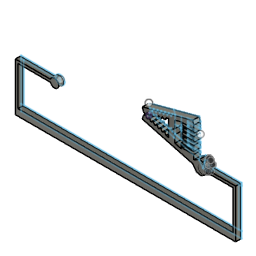
CompliantHands v2 (Autodesk Fusion 360 design; units mm, degrees)
Autodesk Fusion 360 part; units mm, degrees
sketch "Sketch1" plane through (0, 0, 0) normal (0, 1, 0) x (1, 0, 0)
  line L0 (0, 0) -> (19.3185, 5.1764)
  line L1 (0, 0) -> (0.7765, -2.8978)
  line L2 (20.095, 2.2786) -> (19.3185, 5.1764)
  line L3 (0.7765, -2.8978) -> (3.6742, -2.1213)
  line L4 (3.6742, -2.1213) -> (6.572, -1.3449)
  line L5 (6.572, -1.3449) -> (9.4698, -0.5684)
  line L6 (9.4698, -0.5684) -> (12.3676, 0.2081)
  line L7 (12.3676, 0.2081) -> (15.2653, 0.9845)
  line L8 (15.2653, 0.9845) -> (18.1631, 1.761)
  line L9 (0.7765, -2.8978) -> (2.6136, -3.9584)
  line L10 (2.6136, -3.9584) -> (3.6742, -2.1213)
  line L11 (3.6742, -2.1213) -> (5.5114, -3.182)
  line L12 (5.5114, -3.182) -> (6.572, -1.3449)
  line L13 (6.572, -1.3449) -> (8.4091, -2.4055)
  line L14 (8.4091, -2.4055) -> (9.4698, -0.5684)
  line L15 (9.4698, -0.5684) -> (11.3069, -1.6291)
  line L16 (11.3069, -1.6291) -> (12.3676, 0.2081)
  line L17 (12.3676, 0.2081) -> (14.2047, -0.8526)
  line L18 (14.2047, -0.8526) -> (15.2653, 0.9845)
  line L19 (15.2653, 0.9845) -> (17.1025, -0.0762)
  line L20 (17.1025, -0.0762) -> (18.1631, 1.761)
  line L21 (20.095, 2.2786) -> (18.1631, 1.761)
  line L22 (12.3676, -8.3553) -> (15.2653, -9.1317)
  line L23 (9.4698, -7.5788) -> (12.3676, -8.3553)
  line L24 (9.4698, -7.5788) -> (11.3069, -6.5182)
  line L25 (8.4091, -5.7417) -> (9.4698, -7.5788)
  line L26 (6.572, -6.8024) -> (8.4091, -5.7417)
  line L27 (5.5114, -4.9653) -> (6.572, -6.8024)
  line L28 (3.6742, -6.0259) -> (5.5114, -4.9653)
  line L29 (0.7765, -5.2495) -> (2.6136, -4.1888)
  line L30 (2.6136, -4.1888) -> (3.6742, -6.0259)
  line L31 (11.3069, -6.5182) -> (12.3676, -8.3553)
  line L32 (12.3676, -8.3553) -> (14.2047, -7.2946)
  line L33 (14.2047, -7.2946) -> (15.2653, -9.1317)
  line L34 (15.2653, -9.1317) -> (17.1025, -8.0711)
  line L35 (15.2653, -9.1317) -> (18.1631, -9.9082)
  line L36 (17.1025, -8.0711) -> (18.1631, -9.9082)
  line L37 (0, -8.1472) -> (19.3185, -13.3236)
  line L38 (0, -8.1472) -> (0.7765, -5.2495)
  line L39 (0.7765, -5.2495) -> (3.6742, -6.0259)
  line L40 (6.572, -6.8024) -> (9.4698, -7.5788)
  line L41 (3.6742, -6.0259) -> (6.572, -6.8024)
  line L42 (20.095, -10.4258) -> (18.1631, -9.9082)
  line L43 (20.095, -10.4258) -> (19.3185, -13.3236)
  line L44 (20.095, 2.2786) -> (20.095, -10.4258)
  line L45 (19.3185, 5.1764) -> (38.637, 10.3528)
  line L46 (20.095, 2.2786) -> (39.4135, 7.455)
  line L47 (39.4135, 7.455) -> (38.637, 10.3528)
  line L48 (20.095, -10.4258) -> (39.4135, -15.6022)
  line L49 (19.3185, -13.3236) -> (38.637, -18.5)
  line L50 (38.637, -18.5) -> (39.4135, -15.6022)
  line L51 (20.095, 2.2786) -> (24.9246, 3.5727)
  line L52 (24.9246, 3.5727) -> (24.9246, -4.0736)
  line L53 (24.9246, -4.0736) -> (24.9246, -11.7199)
  line L54 (20.095, -4.0736) -> (22.095, -4.0736)
  line L55 (24.9246, -4.0736) -> (24.9246, -6.0736)
  line L56 (22.095, -4.0736) -> (24.9246, -6.0736)
  line L57 (24.9246, -4.0736) -> (24.9246, -2.0736)
  line L58 (22.095, -4.0736) -> (24.9246, -2.0736)
  line L59 (39.4135, 7.455) -> (39.4135, 4.8668)
  line L60 (39.4135, 4.8668) -> (29.7542, 4.8668)
  line L61 (39.4135, -15.6022) -> (39.4135, -13.014)
  line L62 (39.4135, -13.014) -> (29.7542, -13.014)
  line L63 (39.4135, 7.455) -> (43.713, 4.9027)
  line L64 (38.637, 10.3528) -> (41.5877, 14.3893)
  line L65 (41.5877, 14.3893) -> (43.713, 4.9027)
  line L66 (39.4135, 0.8668) -> (38.4135, 0.8668)
  line L67 (39.4135, 0.8668) -> (39.4135, 1.8668)
  line L68 (39.4135, 1.8668) -> (29.7542, 1.8668)
  line L69 (29.7542, 1.8668) -> (29.7542, 0.8668)
  line L70 (29.7542, 0.8668) -> (38.4135, 0.8668)
  line L71 (29.7542, 1.8668) -> (29.7542, 4.8668)
  line L72 (29.7542, 4.8668) -> (30.7542, 4.8668)
  line L73 (30.7542, 4.8668) -> (30.7542, 1.8668)
  line L74 (30.7542, 4.8668) -> (39.4135, 4.8668)
  line L75 (39.4135, 4.8668) -> (39.4135, 5.0729)
  circle A0 centre (45.9703, 10.3897) radius 3.4023
  line L76 (46.28, 5.4777) -> (43.713, 4.9027)
  line L77 (41.5877, 14.3893) -> (44.1548, 14.9643)
  spline S0 degree 5 poles (47.6847, 13.3285) (47.6048, 13.4012) (47.4459, 13.5431) (47.2099, 13.746) (46.8999, 13.9959) (46.5209, 14.2717) (46.1512, 14.5071) (45.7919, 14.6983) (45.4434, 14.8421) (45.106, 14.9387) (44.7788, 14.9908) (44.5247, 14.9995) (44.3382, 14.9886) (44.2156, 14.9737) (44.1548, 14.9643) knots 0 0 0 0 0 0 0.1 0.2 0.3 0.4 0.5 0.6 0.7 0.8 0.9 1 1 1 1 1 1
  spline S1 degree 5 poles (48.7311, 8.4013) (48.6822, 8.304) (48.5842, 8.1125) (48.4374, 7.835) (48.2415, 7.4848) (47.9966, 7.0826) (47.7516, 6.7194) (47.5065, 6.3991) (47.2614, 6.1252) (47.0161, 5.8979) (46.7708, 5.7146) (46.5745, 5.6007) (46.4273, 5.5326) (46.3291, 5.4948) (46.28, 5.4777) knots 0 0 0 0 0 0 0.1 0.2 0.3 0.4 0.5 0.6 0.7 0.8 0.9 1 1 1 1 1 1
  circle A1 centre (45.9703, 10.3897) radius 3.3
  line L78 (45.9703, 10.3897) -> (45.9703, 9.3897)
  line L79 (45.9703, 9.3897) -> (70.9703, 9.3897)
  line L80 (70.9703, 9.3897) -> (70.9703, 10.3897)
  line L81 (45.9703, 10.3897) -> (45.9703, 11.3897)
  line L82 (45.9703, 11.3897) -> (70.9703, 11.3897)
  line L83 (70.9703, 11.3897) -> (70.9703, 10.3897)
  line L84 (39.4135, 4.8668) -> (39.4135, 3.8668)
  line L85 (39.4135, 3.8668) -> (30.7542, 3.8668)
  line L86 (39.4135, 1.8668) -> (39.4135, -1.1332)
  line L87 (39.4135, -1.1332) -> (39.4135, -2.1332)
  line L88 (39.4135, -2.1332) -> (29.7542, -2.1332)
  line L89 (29.7542, -2.1332) -> (29.7542, -1.1332)
  line L90 (29.7542, -1.1332) -> (39.4135, -1.1332)
  line L91 (39.4135, -2.1332) -> (38.4135, -2.1332)
  line L92 (38.4135, -2.1332) -> (38.4135, 0.8668)
  line L93 (29.7542, -2.1332) -> (29.7542, -5.1332)
  line L94 (29.7542, -5.1332) -> (39.4135, -5.1332)
  line L95 (39.4135, -5.1332) -> (39.4135, -4.1332)
  line L96 (39.4135, -4.1332) -> (29.7542, -4.1332)
  line L97 (29.7542, -2.1332) -> (30.7542, -2.1332)
  line L98 (30.7542, -2.1332) -> (30.7542, -5.1332)
  line L99 (39.4135, -5.1332) -> (39.4135, -8.1332)
  line L100 (39.4135, -8.1332) -> (29.7542, -8.1332)
  line L101 (29.7542, -8.1332) -> (29.7542, -7.1332)
  line L102 (29.7542, -7.1332) -> (39.4135, -7.1332)
  line L103 (39.4135, -5.1332) -> (38.4135, -5.1332)
  line L104 (38.4135, -5.1332) -> (38.4135, -7.1332)
  line L105 (29.7542, -8.1332) -> (29.7542, -11.1332)
  line L106 (29.7542, -11.1332) -> (39.4135, -11.1332)
  line L107 (39.4135, -11.1332) -> (39.4135, -10.1332)
  line L108 (39.4135, -10.1332) -> (29.7542, -10.1332)
  line L109 (29.7542, -8.1332) -> (30.7542, -8.1332)
  line L110 (30.7542, -8.1332) -> (30.7542, -10.1332)
  line L111 (39.4135, -11.1332) -> (39.4135, -13.014)
  line L112 (39.4135, -11.1332) -> (38.4135, -11.1332)
  line L113 (38.4135, -11.1332) -> (38.4135, -13.014)
  line L114 (70.9703, 11.3897) -> (70.9703, 41.3897)
  line L115 (70.9703, 41.3897) -> (68.9703, 41.3897)
  line L116 (68.9703, 41.3897) -> (68.9703, 11.3897)
  line L117 (-98.0297, 41.3897) -> (-98.0297, 46.3897)
  line L118 (-98.0297, 46.3897) -> (70.9703, 46.3897)
  line L119 (70.9703, 46.3897) -> (70.9703, 41.3897)
  line L120 (-98.0297, 41.3897) -> (-98.0297, 11.3897)
  line L121 (68.9703, 41.3897) -> (-98.0297, 41.3897)
  line L122 (-98.0297, 11.3897) -> (-96.0297, 11.3897)
  line L123 (-96.0297, 11.3897) -> (-96.0297, 41.3897)
  line L124 (-98.0297, 11.3897) -> (-98.0297, 9.3897)
  line L125 (-98.0297, 9.3897) -> (-68.0297, 9.3897)
  line L126 (-68.0297, 9.3897) -> (-68.0297, 11.3897)
  line L127 (-68.0297, 11.3897) -> (-96.0297, 11.3897)
  circle A2 centre (-68.0297, 10.3897) radius 3.3
  point P0 (45.6581, 14.7479)
  point P1 (47.3897, 6.2744)
  dimension "d1" = 20
  dimension "d2" = 3
  dimension "d3" = 3
  dimension "d4" = 3
  dimension "d5" = 3
  dimension "d6" = 3
  dimension "d7" = 3
  dimension "d8" = 3
  dimension "d15" = 20
  dimension "d16" = 3
  dimension "d17" = 3
  dimension "d18" = 3
  dimension "d19" = 3
  dimension "d20" = 3
  dimension "d21" = 3
  dimension "d22" = 3
  dimension "d23" = 20
  dimension "d24" = 20
  dimension "d26" = 20
  dimension "d27" = 5
  dimension "d28" = 2
  dimension "d29" = 2
  dimension "d30" = 2
  dimension "d51" = 5
  dimension "d52" = 5
  dimension "d59" = 1
  dimension "d60" = 3
  dimension "d61" = 1
  dimension "d67" = 6.6
  dimension "d68" = 25
  dimension "d69" = 1
  dimension "d70" = 1
  dimension "d83" = 1
  dimension "d84" = 3
  dimension "d85" = 1
  dimension "d86" = 1
  dimension "d87" = 1
  dimension "d88" = 3
  dimension "d89" = 1
  dimension "d90" = 1
  dimension "d91" = 3
  dimension "d92" = 1
  dimension "d93" = 1
  dimension "d94" = 3
  dimension "d95" = 1
  dimension "d96" = 1
  dimension "d97" = 1
  dimension "d98" = 30
  dimension "d99" = 2
  dimension "d101" = 5
  dimension "d102" = 2
  dimension "d103" = 2
  dimension "d104" = 30
  dimension "d105" = 2
  dimension "d106" = 6.6
  constraint coincident L0.start L1.start
  constraint perpendicular L0 L1
  constraint perpendicular L0 L2
  constraint perpendicular L1 L3
  constraint perpendicular L1 L4
  constraint perpendicular L2 L21
  constraint perpendicular L37 L38
  constraint perpendicular L37 L43
  constraint perpendicular L38 L39
  constraint perpendicular L38 L41
  constraint perpendicular L42 L43
  constraint vertical L44
  constraint perpendicular L2 L45
  constraint perpendicular L2 L46
  constraint perpendicular L43 L48
  constraint perpendicular L43 L49
  constraint perpendicular L48 L50
  constraint perpendicular L2 L51
  constraint parallel L44 L52
  constraint coincident L48 L53.end
  constraint parallel L52 L53
  constraint midpoint L44 L54.start
  constraint perpendicular L44 L54
  constraint parallel L53 L55
  constraint coincident L52 L57.end
  constraint parallel L57 L59
  constraint midpoint L46 L60.end
  constraint perpendicular L59 L60
  constraint perpendicular L60 L61
  constraint midpoint L48 L62.end
  constraint perpendicular L61 L62
  constraint perpendicular L66 L67
  constraint perpendicular L68 L69
  constraint perpendicular L68 L71
  constraint perpendicular L69 L72
  constraint coincident L68 L73.end
  constraint perpendicular L68 L73
  constraint perpendicular L59 L74
  constraint coincident L59 L75.end
  constraint perpendicular L60 L75
  constraint coincident A0 S1.start
  constraint coincident A0 S0.start
  constraint perpendicular L65 L76
  constraint concentric A0 A1
  constraint coincident A0.centre A1.centre
  constraint perpendicular L78 L79
  constraint perpendicular L80 L82
  constraint perpendicular L60 L84
  constraint coincident L73 L85.end
  constraint perpendicular L73 L85
  constraint perpendicular L68 L86
  constraint perpendicular L68 L87
  constraint perpendicular L69 L88
  constraint perpendicular L70 L89
  constraint perpendicular L87 L90
  constraint coincident L88 L91.end
  constraint perpendicular L70 L92
  constraint perpendicular L88 L93
  constraint perpendicular L87 L94
  constraint perpendicular L91 L95
  constraint coincident L93 L96.end
  constraint perpendicular L93 L96
  constraint perpendicular L93 L97
  constraint coincident L94 L98.end
  constraint perpendicular L94 L98
  constraint perpendicular L94 L99
  constraint perpendicular L95 L100
  constraint perpendicular L100 L101
  constraint perpendicular L95 L102
  constraint perpendicular L99 L103
  constraint coincident L102 L104.end
  constraint perpendicular L102 L104
  constraint perpendicular L100 L105
  constraint perpendicular L105 L106
  constraint perpendicular L100 L107
  constraint coincident L105 L108.end
  constraint perpendicular L105 L108
  constraint perpendicular L101 L109
  constraint coincident L108 L110.end
  constraint perpendicular L108 L110
  constraint perpendicular L62 L111
  constraint perpendicular L111 L112
  constraint coincident L62 L113.end
  constraint perpendicular L62 L113
  constraint perpendicular L82 L114
  constraint perpendicular L114 L115
  constraint coincident L82 L116.end
  constraint perpendicular L82 L116
  constraint vertical L117
  constraint horizontal L118
  constraint vertical L119
  constraint perpendicular L120 L121
  constraint perpendicular L120 L122
  constraint coincident L121 L123.end
  constraint perpendicular L121 L123
  constraint perpendicular L122 L124
  constraint perpendicular L124 L125
  constraint perpendicular L125 L126
  measures "d1" distance of L0.start L0.end
  measures "d2" distance of L0.start L1.end
  measures "d3" distance of L1.end L3.end
  measures "d4" distance of L3.end L4.end
  measures "d5" distance of L4.end L5.end
  measures "d6" distance of L5.end L6.end
  measures "d7" distance of L6.end L7.end
  measures "d8" distance of L7.end L8.end
  measures "d15" distance of L37.start L37.end
  measures "d16" distance of L37.start L29.start
  measures "d17" distance of L29.start L28.start
  measures "d18" distance of L28.start L26.start
  measures "d19" distance of L23.start L26.start
  measures "d20" distance of L22.start L23.start
  measures "d21" distance of L22.end L22.start
  measures "d22" distance of L22.end L35.end
  measures "d23" distance of L0.end L45.end
  measures "d24" distance of L2.start L46.end
  measures "d26" distance of L37.end L49.end
  measures "d27" distance of L2.start L51.end
  measures "d28" distance of L54.start L54.end
  measures "d29" distance of L52.end L55.end
  measures "d30" distance of L52.end L57.end
  measures "d51" distance of L46.end L63.end
  measures "d52" distance of L45.end L64.end
  measures "d59" distance of L66.start L67.end
  measures "d60" distance of L68.end L60.end
  measures "d61" distance of L60.end L72.end
  measures "d67" diameter of A1
  measures "d68" distance of A0.centre L80.end
  measures "d69" distance of A0.centre L78.end
  measures "d70" distance of A0.centre L81.end
  measures "d83" distance of L59.end L84.end
  measures "d84" distance of L67.end L86.end
  measures "d85" distance of L86.end L87.end
  measures "d86" distance of L88.end L89.end
  measures "d87" distance of L87.end L91.end
  measures "d88" distance of L88.end L93.end
  measures "d89" distance of L94.end L95.end
  measures "d90" distance of L88.end L97.end
  measures "d91" distance of L94.end L99.end
  measures "d92" distance of L100.end L101.end
  measures "d93" distance of L94.end L103.end
  measures "d94" distance of L100.end L105.end
  measures "d95" distance of L106.end L107.end
  measures "d96" distance of L100.end L109.end
  measures "d97" distance of L106.end L112.end
  measures "d98" distance of L82.end L114.end
  measures "d99" distance of L114.end L115.end
  measures "d101" distance of L114.end L118.end
  measures "d102" distance of L120.end L122.end
  measures "d103" distance of L120.end L124.end
  measures "d104" distance of L124.end L125.end
  measures "d105" distance of L125.end L126.end
  measures "d106" diameter of A2
extrude "Extrude1" add sketch "Sketch1" against normal blind 5 contours L0 L1 L2 L3 L4 L5 L6 L7 L8 L21 | L2 L45 L46 L47 L51 | L3 L9 L10 | L44 L46 L51 L52 L54 L58 | L4 L11 L12 | L8 L19 L20 | L44 L48 L53 L54 L56 | L46 L59 L60 L72 L74 L75 | L5 L13 L14 | L7 L17 L18 | L22 L23 L35 L37 L38 L39 L40 L41 L42 L43 | L43 L48 L49 L50 | L60 L68 L71 L72 L73 | L6 L15 L16 | L34 L35 L36 | L60 L73 L74 L84 L85 | L66 L67 L68 L69 L70 L86 | L22 L32 L33 | L48 L61 L62 | L23 L24 L31 | L29 L30 L39 | L62 L106 L111 L112 L113 | L66 L86 L90 L92 | L25 L26 L40 | L27 L28 L41 | L105 L106 L107 L108 L112 | L88 L89 L90 L92 L97 | L87 L88 L90 L91 L92 | L100 L105 L108 L109 L110 | L88 L93 L96 L97 L98 | L99 L100 L101 L102 L109 | L93 L94 L96 L98 | L94 L95 L96 L98 L103 | L94 L99 L102 L103 L104 makes body 1
extrude "Extrude2" add sketch "Sketch1" against normal blind 5 contours L47 L63 L64 L65 | L65 A0 L77 S0 | L65 A0 L76 S1 bodies 1
extrude "Extrude3" add sketch "Sketch1" against normal blind 0.5 contours A0 A1 L79 L82 | A0 A1 L79 L82 | A1 L78 L79 L81 L82 | A1 L78 L79 L81 L82 bodies 1
extrude "Extrude4" add sketch "Sketch1" along normal blind -5 and the other way blind 4.5 contours A0 A1 L79 L82 | A0 A1 L79 L82 | A1 L78 L79 L81 L82 | A1 L78 L79 L81 L82 bodies 1
extrude "Extrude5" add sketch "Sketch1" along normal blind -4.4 and the other way blind 0.6 separate body contours A0 L79 L80 L82 L83 | A0 A1 L79 L82 | A1 L78 L79 L81 L82 | A1 L78 L79 L81 L82 | L82 L114 L115 L116 | L115 L117 L118 L119 L121 | L120 L121 L122 L123 | L122 L124 L125 L127 A2 | L125 L126 L127 A2 | L125 L126 L127 A2 picked at (49.1795, 11.2806) makes body 2
named bodies: "Clamp"
